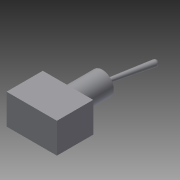
# Autodesk Inventor part: switch
Saved by Autodesk Inventor 2013 SP2 (Build 170200200, 200)
## iProperties
Created: 2018-09-24
Part Number: switch
Material: Generic
Document SubType Name: Modeling
Designer: alex
Density: 1 g/cm^3
Mass: 1.26106 g
Surface Area: 8.28322 cm^2
Volume: 1.26106 cm^3
Author: alex
Autodesk Inventor part; units mm, degrees
ref_plane "YZ Plane" through (0, 0, 0) normal (1, 0, 0) x (0, 1, 0)
ref_plane "XZ Plane" through (0, 0, 0) normal (0, 1, 0) x (-1, 0, 0)
sketch "Sketch1" plane through (0, 0, 0) normal (0, 1, 0) x (-1, 0, 0)
  line L0 (-6.6, -3.95) -> (6.6, -3.95)
  line L1 (6.6, -3.95) -> (6.6, 3.95)
  line L2 (6.6, 3.95) -> (-6.6, 3.95)
  line L3 (-6.6, 3.95) -> (-6.6, -3.95)
  line L4 (-6.6, -3.95) -> (6.6, 3.95) construction
  line L5 (6.6, -3.95) -> (-6.6, 3.95) construction
  point P0 (0, 0)
  dimension "d0" = 13.2
  dimension "d1" = 7.9
  constraints: 12 end point, 2 midpoint, 2 parallel, 1 horizontal, 1 perpendicular
  measures "d0" distance of L2.end L1.end
  measures "d1" distance of L1.end L0.end
extrude "Extrusion1" add sketch "Sketch1" along normal blind 9.5
sketch "Sketch2" plane through (0, 9.5, 0) normal (0, 1, 0) x (1, 0, 0)
  circle A0 centre (0, 0) radius 3
  dimension "d4" = 6
  constraints: 1 centre point, 1 coincident
  measures "d4" diameter of A0
extrude "Extrusion2" add sketch "Sketch2" along normal blind 9
ref_plane "Work Plane1" through (-6.6, 0, 0) normal (0, 0, 1) x (1, 0, 0)
sketch "Sketch3" plane through (-6.6, 0, 0) normal (0, 0, 1) x (1, 0, 0)
  line L0 (9.6, 18.5) -> (3.6, 18.5) projected
  line L1 (3.6, 9.5) -> (9.6, 9.5) projected
  line L2 (6.6, 18.5) -> (9.1507, 30.5)
  arc A0 (9.762, 29.6032) -> (9.1507, 30.5) centre (9.0919, 29.8032) ccw
  line L3 (9.762, 29.6032) -> (7.1, 18.5)
  line L4 (7.1, 18.5) -> (7.0161, 18.1501)
  line L5 (7.0161, 18.1501) -> (6.6, 18.5)
  point P0 (6.6, 0)
  dimension "d8" = 12
  dimension "d9" = 78
  constraints: 8 end point, 2 point on circle, 1 centre point, 1 collinear, 1 midpoint, 1 point on line
  measures "d8" distance from line of L0 L2.end
  measures "d9" angle of L0 L2
revolve "Revolution1" add sketch "Sketch3" angle 360 about axis through (0, 18.5, 0) along (0.2079117, 0.9781476, 0)
body "Solid1"
